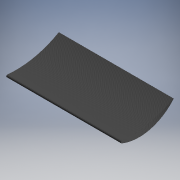
# Autodesk Inventor part: cover
Saved by Autodesk Inventor 2018.1 (Build 221171000, 171)
## iProperties
Created: 2017-10-22
Part Number: cover
Material: CFRP
Document SubType Name: Modeling
Designer: ku_sk
Mass: 134.013 g
Surface Area: 18745.1 cm^2
Volume: 93.7157 cm^3
Density: 1.43 g/cm^3
Appearance: カーボンファイバー
Author: ku_sk
Autodesk Inventor part; units mm, degrees
ref_plane "YZ Plane" through (0, 0, 0) normal (1, 0, 0) x (0, 1, 0)
ref_plane "XZ Plane" through (0, 0, 0) normal (0, 1, 0) x (-1, 0, 0)
ref_plane "XY Plane" through (0, 0, 0) normal (0, 0, 1) x (1, 0, 0)
sketch "スケッチ1" plane through (0, 0, 0) normal (1, 0, 0) x (0, 1, 0)
  line L0 (0, 250) -> (88.1635, -250)
  arc A0 (0, 250) -> (88.1635, -250) centre (710.7652, 117.5543) ccw
  arc A1 (0, 250) -> (88.1635, -250) centre (325.1936, 49.5676) ccw
  line L1 (0, -370.1192) -> (0, 353.3532) projected
  point P0 (0, 0)
  dimension "d0" = 250
  dimension "d2" = 500
  dimension "d3" = 10
  dimension "d4" = 723
  dimension "d5" = 382
  constraints: 4 point on circle, 2 centre point, 2 end point, 1 point on line
  measures "d0" distance of L0.start point (0, 0)
  measures "d2" vertical distance of L0.start L0.end
  measures "d3" angle of L1 L0
  measures "d4" radius of A0
  measures "d5" radius of A1
extrude "押し出し1" add sketch "スケッチ1" along normal mid plane 970 contours A0 L1 A1 | A1 L1 A0
fillet "フィレット1" radius 10 1 edges at (0, 0, 250)
fillet "フィレット2" radius 2 1 edges at (0, 88.1635, -250)
shell "シェル1" thickness 0.1 outward yes removed faces 2 at (485, -17.1174, -13.9662) at (-485, -17.1174, -13.9662)
